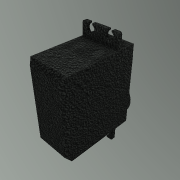
# Autodesk Inventor part: MG996R
Saved by Autodesk Inventor 2015 SP2 (Build 190223200, 223)
## iProperties
Created: 2015-10-08
Part Number: MG996R
Material: Generic
Document SubType Name: Modeling
Designer: styku
Density: 1 g/cm^3
Appearance: Black Cast
Mass: 30.8086 g
Surface Area: 66.8648 cm^2
Volume: 30.8086 cm^3
Author: styku
Autodesk Inventor part; units mm, degrees
ref_plane "YZ Plane" through (0, 0, 0) normal (1, 0, 0) x (0, 1, 0)
ref_plane "XZ Plane" through (0, 0, 0) normal (0, 1, 0) x (-1, 0, 0)
ref_plane "XY Plane" through (0, 0, 0) normal (0, 0, 1) x (1, 0, 0)
sketch "Sketch1" plane through (0, 0, 0) normal (0, 1, 0) x (-1, 0, 0)
  line L0 (10, 20) -> (-10, 20)
  line L1 (-10, 20) -> (-10, -20)
  line L2 (-10, -20) -> (10, -20)
  line L3 (10, -20) -> (10, 20)
  line L4 (21, 0) -> (-27, 0) construction
  line L5 (0, 26) -> (0, -28) construction
  line L6 (9.5, 20) -> (9.5, 27)
  line L7 (-9.5, 27) -> (-9.5, 20)
  line L8 (0.5, 20) -> (0.5, 27)
  line L9 (-0.5, 27) -> (-0.5, 20)
  arc A0 (4, 26.2656) -> (6, 26.2656) centre (5, 24.25) ccw
  line L10 (6, 27) -> (6, 26.2656)
  line L11 (4, 27) -> (4, 26.2656)
  line L12 (9.5, 27) -> (6, 27)
  arc A1 (-6, 26.2656) -> (-4, 26.2656) centre (-5, 24.25) ccw
  line L13 (-6, 27) -> (-6, 26.2656)
  line L14 (-4, 27) -> (-4, 26.2656)
  line L15 (4, 27) -> (-4, 27)
  line L16 (-6, 27) -> (-9.5, 27)
  line L17 (9.5, -20) -> (9.5, -27)
  line L18 (-9.5, -27) -> (-9.5, -20)
  line L19 (0.5, -20) -> (0.5, -27)
  line L20 (-0.5, -27) -> (-0.5, -20)
  arc A2 (6, -26.2656) -> (4, -26.2656) centre (5, -24.25) ccw
  line L21 (6, -27) -> (6, -26.2656)
  line L22 (4, -27) -> (4, -26.2656)
  line L23 (9.5, -27) -> (6, -27)
  line L24 (-6, -27) -> (-6, -26.2656)
  arc A3 (-4, -26.2656) -> (-6, -26.2656) centre (-5, -24.25) ccw
  line L25 (-4, -27) -> (-4, -26.2656)
  line L26 (4, -27) -> (-4, -27)
  line L27 (-6, -27) -> (-9.5, -27)
  arc A4 (-8.75, -5.1588) -> (8.75, -5.1588) centre (0, -10) ccw
  line L28 (8.75, 14.5) -> (-8.75, 14.5)
  line L29 (8.75, 14.5) -> (8.75, -5.1588)
  line L30 (-8.75, 14.5) -> (-8.75, -5.1588)
  circle A5 centre (0, -10) radius 6.5
  circle A6 centre (0, -10) radius 5
  circle A7 centre (0, -10) radius 3
  line L31 (9.5, -20) -> (-9.5, -20)
  line L32 (0.5, -20) -> (0.5, -27)
  line L33 (-0.5, -27) -> (-0.5, -20)
  point P0 (0, 0)
  dimension "d0" = 20
  dimension "d1" = 40
  dimension "d5" = 20
  dimension "d6" = 10
  dimension "d10" = 19
  dimension "d11" = 0.5
  dimension "d12" = 0.5
  dimension "d13" = 1
  dimension "d14" = 4.5
  dimension "d15" = 4.25
  dimension "d16" = 4.5
  dimension "d17" = 2
  dimension "d18" = 1
  dimension "d19" = 7
  dimension "d20" = 10
  dimension "d21" = 5.5
  dimension "d22" = 1.25
  dimension "d23" = 13
  dimension "d24" = 10
  dimension "d25" = 6
  constraints: 68 end point, 25 symmetric about line, 14 perpendicular, 10 point on circle, 9 point on line, 8 centre point, 5 collinear, 4 parallel, 3 coincident, 2 horizontal, 2 vertical, 1 tangent, 3 other
  measures "d0" distance of L2.end L1.end
  measures "d1" distance of L1.end L0.end
  measures "d5" distance between parallel lines of L4 L0
  measures "d6" distance between parallel lines of L5 L3
  measures "d10" distance between parallel lines of L7 L6
  measures "d11" distance between parallel lines of L6 L3
  measures "d12" distance between parallel lines of L5 L8
  measures "d13" distance between parallel lines of L8 L9
  measures "d14" diameter of A0
  measures "d15" distance from line of L0 A0.centre
  measures "d16" distance from line of A0.centre L6
  measures "d17" distance between parallel lines of L11 L10
  measures "d18" distance from line of A0.centre L10
  measures "d19" distance between parallel lines of L0 L12
  measures "d20" distance from line of L2 A4.centre
  measures "d21" distance between parallel lines of L0 L28
  measures "d22" distance between parallel lines of L3 L29
  measures "d23" diameter of A5
  measures "d24" diameter of A6
  measures "d25" diameter of A7
extrude "Extrusion1" add sketch "Sketch1" along normal blind 1.8 contours L3 A4 L29 L28 L30 L1 L0 | L0 L8 L15 L11 A0 L10 L12 L6 | L3 L2 A4 | A4 L30 L28 L29 | L0 L9 L15 L8 | L2 L19 L26 L20 | L2 L1 A4 | L0 L7 L16 L13 A1 L14 L15 L9 | L17 L23 L21 A2 L22 L26 L19 L2 | L20 L26 L25 A3 L24 L27 L18 L2 | A5 | A6 | A7
extrude "Extrusion2" add sketch "Sketch1" along normal blind 9 contours L3 A4 L29 L28 L30 L1 L0 | L3 L2 A4 | A4 L30 L28 L29 | L2 L1 A4 | A5 | A6 | A7
extrude "Extrusion3" add sketch "Sketch1" along normal blind 11 contours A4 L30 L28 L29
extrude "Extrusion4" cut sketch "Sketch1" along normal blind 12 contours A5
extrude "Extrusion5" add sketch "Sketch1" along normal blind 12 contours A5
extrude "Extrusion6" add sketch "Sketch1" along normal blind 12.5 contours A6
extrude "Extrusion7" cut sketch "Sketch1" along normal blind 17 contours A7
extrude "Extrusion8" add sketch "Sketch1" along normal blind 17 contours A7
extrude "Extrusion9" add sketch "Sketch1" against normal blind 27.5 contours L3 A4 L29 L28 L30 L1 L0 | L3 L2 A4 | A4 L30 L28 L29 | L2 L1 A4 | A5 | A6 | A7
fillet "Fillet1" radius 1 4 edges at (9.5, 0.9, -27) (-9.5, 0.9, -27) (9.5, 0.9, 27) (-9.5, 0.9, 27)
fillet "Fillet2" radius 1 1 edges at (3, 17, -10)
chamfer "Chamfer1" distance 2 angle 45 4 edges at (10, -27.5, 0) (0, -27.5, 20) (-10, -27.5, 0) (0, -27.5, -20)
body "Solid1"
